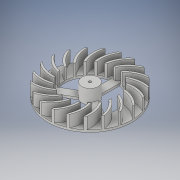
# Autodesk Inventor part: Impeller
Saved by Autodesk Inventor 2017 (Build 210142000, 142)
## iProperties
Created: 2016-08-30
Part Number: Impeller
Material: Generic
Document SubType Name: Modeling
Designer: yash
Density: 1 g/cm^3
Appearance: Default
Author: yash
Autodesk Inventor part; units mm, degrees
ref_plane "YZ Plane" through (0, 0, 0) normal (1, 0, 0) x (0, 1, 0)
ref_plane "XY Plane" through (0, 0, 0) normal (0, 0, 1) x (1, 0, 0)
sketch "Sketch1" plane through (0, 0, 0) normal (0, 1, 0) x (-1, 0, 0)
  circle A0 centre (0, 0) radius 16.2941
  circle A1 centre (0, 0) radius 9.9441
  dimension "d0" = 32.5882
  dimension "d1" = 6.35
  constraints: 2 centre point, 2 coincident
  measures "d0" diameter of A0
  measures "d1" radial gap between concentric circles of A0 A1
extrude "Extrusion1" add sketch "Sketch1" along normal blind 0.8636
sketch "Sketch2" plane through (0, 0.8636, 0) normal (0, 1, 0) x (1, 0, 0)
  arc A0 (-9.9441, 0) -> (-15.094, -6.1374) centre (-5.1376, -9.2625) ccw construction
  line L0 (-9.9441, 0) -> (-15.094, -6.1374) construction
  line L1 (-9.9441, 0) -> (-1.9322, 0) construction
  arc A1 (-9.9065, -0.8636) -> (-14.7134, -7.001) centre (-4.1766, -10.3024) ccw construction
  arc A2 (-15.094, 6.1374) -> (-9.9441, 0) centre (-5.1376, 9.2625) ccw
  arc A3 (-14.7134, 7.001) -> (-9.9065, 0.8636) centre (-4.1766, 10.3024) ccw
  arc A4 (-9.9065, 0.8636) -> (-9.9441, 0) centre (0, 0) ccw
  arc A5 (-14.7134, 7.001) -> (-15.094, 6.1374) centre (0, 0) ccw
  point P0 (-13.1191, -2.54)
  point P1 (-12.2555, -3.4036)
  dimension "d4" = 130
  dimension "d5" = 2.54
  dimension "d6" = 3.175
  dimension "d7" = 0.8636
  dimension "d8" = 0.8636
  dimension "d9" = 0.8636
  dimension "d10" = 0.8636
  dimension "d43" = 16.2941
  dimension "d44" = 9.9441
  dimension "d45" = 11.0419
  constraints: 14 point on circle, 6 centre point, 5 symmetric about line, 4 end point, 2 coincident, 1 equal length, 1 horizontal, 1 horizontal alignment, 2 other
  measures "d4" angle of L0 L1
  measures "d5" vertical distance of L0.start point (-13.119, -2.54)
  measures "d6" horizontal distance of L0.start point (-13.119, -2.54)
  measures "d7" horizontal distance of point (-12.255, -3.404) point (-13.119, -2.54)
  measures "d8" horizontal distance of point (-12.255, -3.404) point (-13.119, -2.54)
  measures "d9" vertical distance of L0.start A1.start
  measures "d10" vertical distance of L0.end A1.end
  measures "d43" radius of A5
  measures "d44" radius of A4
  measures "d45" radius of A3
extrude "Extrusion2" add sketch "Sketch2" along normal blind 4.572
pattern_circular "Circular Pattern1" count 21 over 360 about axis through (0, 0, 0) along (0, 1, 0) of "Extrusion2"
ref_plane "Work Plane1" through (0, 0, 0) normal (0, 1, 0) x (-1, 0, 0)
sketch "Sketch3" plane through (0, 0, 0) normal (0, 1, 0) x (-1, 0, 0)
  circle A0 centre (0, 0) radius 9.9702 construction
  circle A1 centre (0, 0) radius 3.175
  line L0 (1.5875, -2.7496) -> (1.5875, -9.843)
  line L1 (-1.5875, -2.7496) -> (-1.5875, -9.843)
  arc A2 (-1.5875, -9.843) -> (1.5875, -9.843) centre (0, 0) ccw
  circle A3 centre (0, 0) radius 9.9702 construction
  line L2 (1.5875, 2.7496) -> (7.7306, 6.2963)
  line L3 (3.175, 0) -> (9.3181, 3.5467)
  circle A4 centre (0, 0) radius 9.9702 construction
  line L4 (-3.175, 0) -> (-9.3181, 3.5467)
  line L5 (-1.5875, 2.7496) -> (-7.7306, 6.2963)
  dimension "d17" = 6.35
  dimension "d18" = 3.175
  dimension "d19" = 1.5875
  dimension "d22" = 360
  constraints: 12 end point, 10 point on circle, 5 centre point, 5 coincident, 1 parallel, 1 vertical, 23 other
  measures "d17" diameter of A1
  measures "d18" distance between parallel lines of L0 L1
  measures "d19" distance from line of point (0, 0) L1
extrude "Extrusion3" add sketch "Sketch3" along normal blind 5.4864 contours A1
sketch "Sketch4" plane through (0, 5.4864, 0) normal (0, 1, 0) x (1, 0, 0)
  point P0 (0, 0)
  point P1 (0, 0)
  constraints: 1 coincident
hole "Hole1" at (0, 5.4864, 0) direction (0, -1, 0) diameter 1 end through all
sketch "Sketch5" plane through (0, 0, 0) normal (0, 1, 0) x (-1, 0, 0)
  line L0 (1.5875, -2.4015) -> (1.5875, -9.8166)
  line L1 (-1.5875, -2.6189) -> (-1.5875, -9.8166)
  circle A0 centre (0, 0) radius 9.9441 projected
  circle A1 centre (0, 0) radius 9.9441 projected
  arc A2 (-1.5875, -2.6189) -> (1.5875, -2.6189) centre (0, 0) ccw
  arc A3 (-1.5875, -9.8166) -> (1.5875, -9.8166) centre (0, 0) ccw
  line L2 (1.286, 2.5756) -> (7.7076, 6.2831)
  line L3 (3.0618, -0.0653) -> (9.2951, 3.5335)
  arc A4 (9.2951, 3.5335) -> (7.7076, 6.2831) centre (0, 0) ccw
  arc A5 (3.0618, -0.0653) -> (1.4743, 2.6843) centre (0, 0) ccw
  line L4 (-2.8735, -0.1741) -> (-9.2951, 3.5335)
  line L5 (-1.4743, 2.6843) -> (-7.7076, 6.2831)
  arc A6 (-7.7076, 6.2831) -> (-9.2951, 3.5335) centre (0, 0) ccw
  arc A7 (-1.4743, 2.6843) -> (-3.0618, -0.0653) centre (0, 0) ccw
  point P0 (0, -9.9441)
  point P1 (-2.9932, -9.4829)
  point P2 (3.8054, -9.1872)
  point P3 (0.8636, -9.9065)
  dimension "d33" = 3.175
  dimension "d34" = 1.5875
  dimension "d35" = 7.4151
  dimension "d36" = 7.1976
  dimension "d39" = 360
  constraints: 14 point on circle, 12 end point, 6 centre point, 4 coincident, 3 point on line, 1 parallel, 1 vertical, 34 other
  measures "d33" distance between parallel lines of L0 L1
  measures "d34" distance from line of point (0, 0) L1
  measures "d35" distance of L0.start L0.end
  measures "d36" distance of L1.start L1.end
extrude "Extrusion4" add sketch "Sketch5" along normal blind 0.8636 contours L0 A0 L1 A2 | A0 L5 A7 L4 | L3 A5 L2 A0
body "Solid1"
